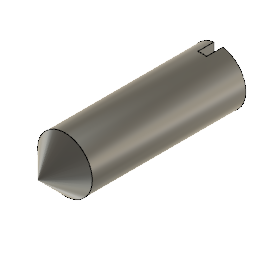
_set screw.b4d3e496-58ed-40b8-ac61-1f8405dbb25f (Autodesk Fusion 360 design; units mm, degrees)
Autodesk Fusion 360 part; units mm, degrees
sketch "Sketch1" plane through (0, 0, 0) normal (0, 1, 0) x (1, 0, 0)
  circle A0 centre (0, 0) radius 5
  dimension "d1" = 10
  constraint coincident A0.centre origin
  measures "d1" diameter of A0
extrude "Extrude1" add sketch "Sketch1" along normal blind 33
chamfer "Chamfer1" distance 5 angle 45 1 edges at (-4.6616, 0, 1.8081)
ref_plane "WorkPlane1" through (0, 0, -5) normal (0, 0, 1) x (1, 0, 0)
sketch "Sketch2" plane through (0, 0, -5) normal (0, 0, 1) x (1, 0, 0)
sketch "Sketch3" plane through (0, 33, 0) normal (0, 1, 0) x (-1, 0, 0)
  circle A0 centre (0, 0) radius 5
  line L0 (0, 0) -> (0.8, 0)
  line L1 (0, 0) -> (-0.8, 0)
  line L2 (-0.8, 0) -> (-0.8, 5.3819)
  line L3 (0.8, 0) -> (0.8, 5.3174)
  line L4 (0.8, 5.3174) -> (-0.8, 5.3819)
  line L5 (0.8, 0) -> (0.8, -5.6853)
  line L6 (-0.8, 0) -> (-0.8, -5.7176)
  line L7 (-0.8, -5.7176) -> (0.8, -5.6853)
  dimension "d6" = 0.8
  dimension "d7" = 0.8
  constraint coincident A0.centre L0.start
  constraint horizontal L0
  constraint parallel L0 L1
  constraint perpendicular L1 L2
  constraint perpendicular L0 L3
  constraint perpendicular L0 L5
  constraint perpendicular L1 L6
  measures "d6" distance of A0.centre L0.end
  measures "d7" distance of A0.centre L1.end
extrude "Extrude2" cut sketch "Sketch3" against normal blind 3 contours A0 L0 L1 L2 L3 | A0 L0 L1 L5 L6
